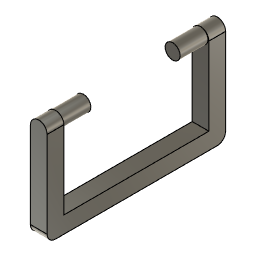
Ensamble dron BPI v17 (Autodesk Fusion 360 archive; units mm, degrees)
design "soporte bateria"
Autodesk Fusion 360 part; units mm, degrees
sketch "Sketch6" plane through (0, 0, 0) normal (0, 0, 1) x (1, 0, 0)
  line L0 (0, 0) -> (3, 0)
  line L1 (3, 0) -> (3, 26)
  line L2 (3, 26) -> (0, 26)
  line L3 (0, 26) -> (0, 0)
  dimension "d27" = 3
  dimension "d28" = 26
  constraint horizontal L0
  constraint vertical L1
  constraint horizontal L2
  constraint vertical L3
  constraint coincident L0.start L3.end
  measures "d27" distance of L0.start L0.end
  measures "d28" distance of L0.start L2.end
extrude "Extrude8" add sketch "Sketch6" along normal blind 3
sketch "Sketch7" plane through (0, 0, 0) normal (0, 1, 0) x (1, 0, 0)
sketch "Sketch8" plane through (0, 0, 0) normal (0, -1, 0) x (1, 0, 0)
  line L0 (0, 0) -> (3, 0)
  line L1 (3, 0) -> (3, 3)
  line L2 (3, 3) -> (0, 3)
  line L3 (0, 3) -> (0, 0)
  line L4 (3, 3) -> (0, 3)
  line L5 (0, 3) -> (0, 18.5)
  line L6 (0, 18.5) -> (3, 18.5)
  line L7 (3, 18.5) -> (3, 3)
  dimension "d31" = 3
  dimension "d32" = 15.5
  constraint horizontal L4
  constraint vertical L5
  constraint horizontal L6
  constraint vertical L7
  constraint coincident L1.end L2.start
  measures "d31" distance of L1.end L2.end
  measures "d32" distance of L1.end L6.end
extrude "Extrude9" add sketch "Sketch8" along normal blind 3
sketch "Sketch9" plane through (0, 26, 0) normal (0, 1, 0) x (-1, 0, 0)
  line L0 (-3, 0) -> (0, 0)
  line L1 (0, 0) -> (0, 3)
  line L2 (0, 3) -> (-3, 3)
  line L3 (-3, 3) -> (-3, 0)
  line L4 (0, 0) -> (-3, 0)
  line L5 (-3, 0) -> (-3, 18.5)
  line L6 (-3, 18.5) -> (0, 18.5)
  line L7 (0, 18.5) -> (0, 0)
  dimension "d35" = 3
  dimension "d36" = 18.5
  constraint horizontal L4
  constraint vertical L5
  constraint horizontal L6
  constraint vertical L7
  constraint coincident L0.end L1.start
  measures "d35" distance of L0.end L0.start
  measures "d36" distance of L0.end L6.end
extrude "Extrude10" add sketch "Sketch9" along normal blind 3
sketch "Sketch10" plane through (0, 0, 0) normal (0, 1, 0) x (-1, 0, 0)
  line L0 (-3, 3) -> (0, 3)
  line L1 (0, 3) -> (0, 18.5)
  line L2 (0, 18.5) -> (-3, 18.5)
  line L3 (-3, 18.5) -> (-3, 3)
  line L4 (-1.5, 18.5) -> (-1.5, 17)
  circle A0 centre (-1.5, 17) radius 1.5
  dimension "d39" = 1.5
  dimension "d40" = 3
  constraint midpoint L2 L4.start
  constraint perpendicular L2 L4
  constraint coincident L4.end A0.centre
  measures "d39" distance of L4.start L4.end
  measures "d40" diameter of A0
sketch "Sketch12" plane through (0, 26, 0) normal (0, -1, 0) x (1, 0, 0)
  line L0 (0, 3) -> (3, 3)
  line L1 (3, 3) -> (3, 18.5)
  line L2 (3, 18.5) -> (0, 18.5)
  line L3 (0, 18.5) -> (0, 3)
  line L4 (1.5, 18.5) -> (1.5, 17.15)
  circle A0 centre (1.5, 17.15) radius 1.35
  dimension "d53" = 1.35
  dimension "d54" = 2.7
  constraint midpoint L2 L4.start
  constraint perpendicular L2 L4
  constraint coincident L4.end A0.centre
  measures "d53" distance of L4.start L4.end
  measures "d54" diameter of A0
extrude "Extrude15" add sketch "Sketch12" along normal blind 5 contours A0
sketch "Sketch13" plane through (0, 0, 0) normal (0, 1, 0) x (-1, 0, 0)
  line L0 (-3, 3) -> (0, 3)
  line L1 (0, 3) -> (0, 18.5)
  line L2 (0, 18.5) -> (-3, 18.5)
  line L3 (-3, 18.5) -> (-3, 3)
  line L4 (-1.5, 18.5) -> (-1.5, 17.15)
  circle A0 centre (-1.5, 17.15) radius 1.35
  dimension "d57" = 1.35
  dimension "d58" = 2.7
  constraint midpoint L2 L4.start
  constraint perpendicular L2 L4
  constraint coincident L4.end A0.centre
  measures "d57" distance of L4.start L4.end
  measures "d58" diameter of A0
extrude "Extrude16" add sketch "Sketch13" along normal blind 5 contours A0
fillet "Fillet4" radius 1.5 8 edges at (3, -1.5, 18.5) (1.5, -3, 18.5) (0, -1.5, 18.5) (1.5, 29, 18.5) (3, 27.5, 18.5) (0, 27.5, 18.5) (1.5, 29, 0) (1.5, -3, 0)
